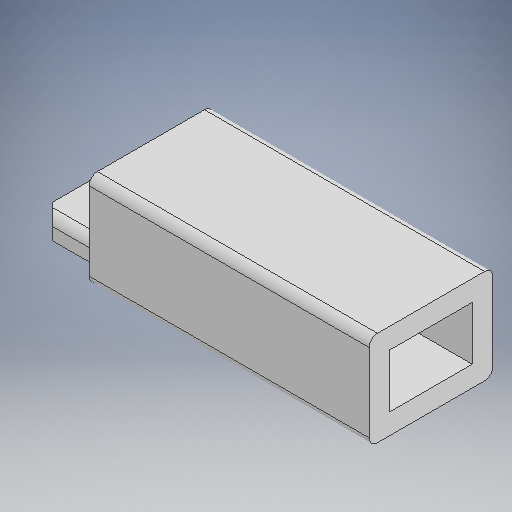
# Autodesk Inventor part: camsera_case_girl
Saved by Autodesk Inventor 2025.2 (Build 292293000, 293)
## iProperties
Created: 2025-03-10
Part Number: camsera_case_girl
Material: 일반
Document SubType Name: Modeling
Designer: jbhma
Density: 1 g/cm^3
Appearance: 기본값
Author: jbhma
Autodesk Inventor part; units mm, degrees
ref_plane "YZ Plane" through (0, 0, 0) normal (1, 0, 0) x (0, 1, 0)
ref_plane "XZ Plane" through (0, 0, 0) normal (0, 1, 0) x (-1, 0, 0)
ref_plane "XY Plane" through (0, 0, 0) normal (0, 0, 1) x (1, 0, 0)
sketch "스케치12" plane through (0, 0, 0) normal (0, 1, 0) x (-1, 0, 0)
  line L0 (0, 0) -> (-63, 0)
  line L1 (-63, 0) -> (-63, -20)
  line L2 (-63, -20) -> (0, -20)
  line L3 (0, -20) -> (0, 0)
  dimension "d57" = 63
  dimension "d58" = 20
  constraints: 8 end point, 2 parallel, 1 horizontal, 1 perpendicular
  measures "d57" distance of L2.end L1.end
  measures "d58" distance of L1.end L0.end
extrude "돌출9" add sketch "스케치12" along normal blind 5
sketch "스케치13" plane through (0, 0, 0) normal (0, -1, 0) x (1, 0, 0)
  line L0 (0, 0) -> (63, 0)
  line L1 (63, 0) -> (63, 5)
  line L2 (63, 5) -> (0, 5)
  line L3 (0, 5) -> (0, 0)
  line L4 (0, -20) -> (63, -20)
  line L5 (63, -20) -> (63, -25)
  line L6 (63, -25) -> (0, -25)
  line L7 (0, -25) -> (0, -20)
  line L8 (0, -25) -> (-5, -25)
  line L9 (-5, -25) -> (-5, 5)
  line L10 (-5, 5) -> (0, 5)
  line L11 (0, 5) -> (0, -25)
  dimension "d61" = 63
  dimension "d62" = 5
  dimension "d63" = 63
  dimension "d64" = 5
  dimension "d65" = 5
  dimension "d66" = 30
  constraints: 24 end point, 6 parallel, 3 horizontal, 3 perpendicular
  measures "d61" distance of L2.end L1.end
  measures "d62" distance of L1.end L0.end
  measures "d63" distance of L5.end L6.end
  measures "d64" distance of L4.end L5.end
  measures "d65" distance of L9.end L10.end
  measures "d66" distance of L8.end L9.end
extrude "돌출10" add sketch "스케치13" against normal blind 28
sketch "스케치15" plane through (-5, 0, -25) normal (-1, 0, 0) x (0, 0, 1)
  line L0 (0, 28) -> (30, 28)
  line L1 (30, 28) -> (30, 23)
  line L2 (30, 23) -> (0, 23)
  line L3 (0, 23) -> (0, 28)
  point P0 (25, 0)
  constraints: 8 end point, 2 parallel, 1 horizontal, 1 perpendicular
extrude "돌출11" cut sketch "스케치15" against normal blind 68
sketch "스케치18" plane through (0, 5, -20) normal (0, 0, 1) x (1, 0, 0)
  line L0 (0, 18) -> (63, 18)
  line L1 (63, 18) -> (63, 13)
  line L2 (63, 13) -> (0, 13)
  line L3 (0, 13) -> (0, 18)
  point P0 (0, -5)
  dimension "d73" = 5
  constraints: 8 end point, 2 parallel, 1 horizontal, 1 perpendicular
  measures "d73" distance of L0.end L1.end
extrude "돌출12" add sketch "스케치18" along normal blind 20
sketch "스케치19" plane through (-5, 0, -25) normal (-1, 0, 0) x (0, 0, 1)
  line L0 (25, 0) -> (5, 0)
  line L1 (5, 0) -> (5, 5)
  line L2 (5, 5) -> (25, 5)
  line L3 (25, 5) -> (25, 0)
  constraints: 8 end point, 2 parallel, 1 horizontal, 1 perpendicular
extrude "돌출13" add sketch "스케치19" along normal blind 17
sketch "스케치20" plane through (-5, 5, 0) normal (0, 1, 0) x (1, 0, 0)
  line L0 (0, 20) -> (-17, 20) projected
  circle A0 centre (-8.5, 10) radius 3.75
  point P0 (5, 0)
  dimension "d79" = 7.5
  dimension "d80" = 10
  constraints: 1 centre point
  measures "d79" diameter of A0
  measures "d80" distance from line of A0.centre L0
extrude "돌출14" cut sketch "스케치20" against normal blind 17
chamfer "모따기1" distance 3 angle 45 2 edges at (-22, 2.5, -20) (-22, 2.5, 0)
fillet "모깎기1" radius 2 2 edges at (29, 23, -25) (29, 23, 5)
fillet "모깎기2" radius 2 1 edges at (-12, 5, 0)
fillet "모깎기3" radius 2 1 edges at (-22, 0, -10)
fillet "모깎기4" radius 2 1 edges at (29, 0, -25)
fillet "모깎기5" radius 2 1 edges at (29, 0, 5)
